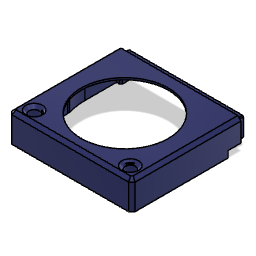
Custom_fan_TeslaK20xm_assembly (Autodesk Fusion 360 archive; units mm, degrees)
design "Case_top"
Autodesk Fusion 360 part; units mm, degrees
note: some values were not read from the file. Set by a fixed rule: which face or edge a step refers to.
sketch "Sketch1" plane through (0, 0, 0) normal (0, 1, 0) x (1, 0, 0)
  line L0 (48, -42.5) -> (-48, -42.5)
  line L1 (-48, -42.5) -> (-48, 42.5)
  line L2 (-48, 42.5) -> (48, 42.5)
  line L3 (48, 42.5) -> (48, -42.5)
  line L4 (48, -42.5) -> (-48, 42.5) construction
  line L5 (-48, -42.5) -> (48, 42.5) construction
  dimension "d1" = 96
  dimension "d2" = 85
  constraint horizontal L0
  constraint perpendicular L0 L1
  constraint parallel L0 L2
  constraint parallel L1 L3
  constraint coincident L4 origin
  constraint coincident L5 origin
  measures "d1" distance of L1.end L2.end
  measures "d2" distance of L0.end L1.end
extrude "Extrude1" add sketch "Sketch1" along normal blind 22.4
sketch "Sketch3" plane through (0, 22.4, 0) normal (0, 1, 0) x (-1, 0, 0)
  line L0 (-48, -42.5) -> (48, -42.5)
  line L1 (48, -42.5) -> (48, 42.5)
  line L2 (48, 42.5) -> (-48, 42.5)
  line L3 (-48, 42.5) -> (-48, -42.5)
  line L4 (48, -42.5) -> (-48, 42.5) construction
  line L5 (-48, -42.5) -> (48, 42.5) construction
  line L6 (0, 0) -> (48, 0) construction
  line L7 (0, 0) -> (0, -42.5) construction
  circle A0 centre (37.4349, 33.1455) radius 4
  circle A1 centre (37.4349, -33.1455) radius 4
  circle A2 centre (-37.4349, -33.1455) radius 4
  circle A3 centre (-37.4349, 33.1455) radius 4
  dimension "d7" = 8
  dimension "d17" = 50
  constraint coincident L0.end L1.start
  constraint coincident L2.end L3.start
  constraint coincident L0.start L3.end
  constraint coincident L1.end L2.start
  constraint coincident L6.start L7.start
  constraint midpoint L1 L6.end
  constraint midpoint L0 L7.end
  constraint coincident L5 A0.centre
  constraint symmetric L6 A0 A1
  constraint symmetric L7 A0 A3
  constraint symmetric L7 A1 A2
  measures "d7" diameter of A0
  measures "d17" distance of L6.start A0.centre
extrude "Extrude2" cut sketch "Sketch3" against normal up to surface (20.9 mm away) contours A0 | A3
chamfer "Chamfer2" distance 2.5 angle 45 2 edges at (-48, 11.2, 42.5) (48, 11.2, 42.5)
sketch "Sketch4" plane through (0, 22.4, 0) normal (0, 1, 0) x (-1, 0, 0)
  line L0 (-48, 40) -> (-48, -42.5)
  line L1 (-48, -42.5) -> (48, -42.5)
  line L2 (48, -42.5) -> (48, 40)
  line L3 (45.5, 42.5) -> (-45.5, 42.5)
  circle A0 centre (37.4349, 33.1455) radius 4
  circle A1 centre (-37.4349, 33.1455) radius 4
  circle A2 centre (0, 0) radius 34
  line L4 (-45.5, 42.5) -> (-48, 40)
  line L5 (48, 40) -> (45.5, 42.5)
  dimension "d11" = 68
  constraint coincident A2.centre origin
  measures "d11" diameter of A2
chamfer "Chamfer1" distance 2.5 angle 45 7 edges at (-48, 22.4, -1.25) (-46.75, 22.4, 41.25) (0, 22.4, 42.5) (46.75, 22.4, 41.25) (48, 22.4, -1.25) (-33.7056, 22.4, 34.592) (41.1642, 22.4, 34.592)
shell "Shell1" thickness 1.5 removed faces 2 at (-15.1667, 0, -14.1667) at (-15.1667, 7.4667, -42.5)
extrude "Extrude3" cut sketch "Sketch4" against normal through all contours A2
sketch "Sketch5" plane through (0, 0, 0) normal (0, -1, 0) x (1, 0, 0)
  circle A0 centre (-37.4349, 33.1455) radius 2.25
  line L0 (0, 0) -> (9, 0) construction
  line L1 (0, 0) -> (0, 1) construction
  line L2 (0, 1) -> (0, 8) construction
  circle A1 centre (37.4349, 33.1455) radius 2.25
  circle A2 centre (37.4349, 33.1455) radius 5.5
  line L3 (46.5, 39.3787) -> (46.5, -42.5)
  line L4 (46.5, -42.5) -> (48, -42.5)
  line L5 (48, -42.5) -> (48, 40)
  line L6 (48, 40) -> (45.5, 42.5)
  line L7 (45.5, 42.5) -> (-45.5, 42.5)
  line L8 (-45.5, 42.5) -> (-48, 40)
  line L9 (-48, 40) -> (-48, -42.5)
  line L10 (-48, -42.5) -> (-46.5, -42.5)
  line L11 (-46.5, -42.5) -> (-46.5, 39.3787)
  line L12 (-46.5, 39.3787) -> (-44.8787, 41)
  line L13 (-44.8787, 41) -> (44.8787, 41)
  line L14 (44.8787, 41) -> (46.5, 39.3787)
  circle A3 centre (-37.4349, 33.1455) radius 5.5
  dimension "d13" = 4.5
  constraint coincident L0.start L1.start
  constraint horizontal L0
  constraint perpendicular L0 L1
  constraint perpendicular L0 L2
  constraint symmetric A0 L2 A1
  measures "d13" diameter of A0
extrude "Extrude4" cut sketch "Sketch5" against normal through all contours A0 | A1
sketch "Sketch6" plane through (0, 0, 0) normal (0, -1, 0) x (1, 0, 0)
  line L0 (46.5, 39.3787) -> (46.5, -42.5)
  line L1 (46.5, -42.5) -> (48, -42.5)
  line L2 (48, -42.5) -> (48, 40)
  line L3 (48, 40) -> (45.5, 42.5)
  line L4 (45.5, 42.5) -> (-45.5, 42.5)
  line L5 (-45.5, 42.5) -> (-48, 40)
  line L6 (-48, 40) -> (-48, -42.5)
  line L7 (-48, -42.5) -> (-46.5, -42.5)
  line L8 (-46.5, -42.5) -> (-46.5, 39.3787)
  line L9 (-46.5, 39.3787) -> (-44.8787, 41)
  line L10 (-44.8787, 41) -> (44.8787, 41)
  line L11 (44.8787, 41) -> (46.5, 39.3787)
  line L12 (48, -42.5) -> (12, -42.5)
  line L13 (12, -42.5) -> (12, -41.1913)
  spline S0 degree 5 poles (14.495, -37.8387) (15.594, -37.5093) (17.7608, -36.7724) (20.9168, -35.4332) (24.9264, -33.1775) (29.5475, -29.5535) (33.7057, -25.1004) (37.3381, -19.8036) (40.4311, -13.6982) (43.0138, -6.8584) (45.1276, 0.6384) (46.4759, 7.1092) (47.3069, 12.2099) (47.7821, 15.7186) (48, 17.5) knots 0 0 0 0 0 0 0.1 0.2 0.3 0.4 0.5 0.6 0.7 0.8 0.9 1 1 1 1 1 1
  line L14 (48, 17.5) -> (48, -42.5)
  arc A0 (14.495, -37.8387) -> (12, -41.1913) centre (15.5, -41.1913) ccw
  line L15 (46.5, -41) -> (13.5092, -41)
  arc A1 (14.9257, -39.2756) -> (13.5092, -41) centre (15.5, -41.1913) ccw
  spline S1 degree 3 poles (14.9257, -39.2756) (22.097, -37.1258) (28.5847, -33.0615) (33.8097, -26.9591) (38.0341, -22.0255) (41.3619, -15.7498) (43.8832, -8.4629) (44.8686, -5.6148) (45.7368, -2.6127) (46.5, 0.5227) knots 0 0 0 0 0.377112 0.377112 0.377112 0.682001 0.682001 0.682001 0.801168 0.801168 0.801168 0.801168
  line L16 (46.5, 0.5227) -> (46.5, -41)
  circle A2 centre (0, 0) radius 44.4282 construction
  arc A3 (44.3977, -1.6437) -> (17.1132, 41) centre (0, 0) ccw
  arc A4 (45.8967, -1.6992) -> (17.691, 42.3843) centre (0, 0) ccw
  arc A5 (-17.1132, 41) -> (-44.4282, 0.0027) centre (0, 0) ccw
  line L17 (-44.8787, 38.7071) -> (-44.8787, -42.5)
  arc A6 (-17.691, 42.3843) -> (-45.9282, 0.0027) centre (0, 0) ccw
  line L18 (-44.4281, 0.0027) -> (-46.5, 0.0027)
  line L19 (-44.4281, 0.0027) -> (-44.4282, -1.4973)
  line L20 (-44.4282, -1.4973) -> (-46.5, -1.4973)
  point P0 (12, -38.5)
  point P1 (35, -23)
  dimension "d21" = 4
  dimension "d22" = 60
  dimension "d23" = 3.5
  dimension "d24" = 1.5
  dimension "d28" = 1.5
  dimension "d29" = 1.5
  dimension "d32" = 1.5
  constraint coincident L1.end L2.start
  constraint perpendicular L2 L12
  constraint perpendicular L12 L13
  constraint coincident L2 S0.end
  constraint perpendicular L1 L14
  constraint coincident P0 L13
  constraint tangent L13 A0
  constraint tangent S0 A0
  constraint coincident A2.centre A3.centre
  constraint coincident A2 A3.end
  constraint coincident S0 A3.start
  constraint coincident A2 A3.start
  constraint coincident L10 A3.end
  constraint coincident A2 L18.start
  constraint coincident A2 A5.start
  constraint coincident L10 A5.start
  constraint horizontal L18
  constraint tangent A2 L19
  constraint coincident L8 L20.end
  constraint perpendicular L8 L20
  measures "d21" distance of L12.end P0
  measures "d22" distance of L1.end S0.end
  measures "d23" radius of A0
  measures "d32" vertical distance of L18.start L19.end
extrude "Extrude6" add sketch "Sketch6" against normal up to surface (20.9 mm away) contours L10 S0 A3 A4 | L10 A5 L17 A6 L18
extrude "Extrude5" add sketch "Sketch6" against normal up to surface (20.9 mm away) contours L0 L12 L13 S0 A0 L15 A1 S1 | L17 L18 L19 L20 | L8 L17 L18 L20
fillet "Fillet3" radius 48 1 edges at (-46.5, 9.6393, -1.4973)
fillet "Fillet4" radius 20 3 edges at (-17.1132, 9.6393, 41) (17.1132, 9.6393, 41) (44.3977, 10.45, -1.6437)
sketch "Sketch7" plane through (48, 0, 0) normal (1, 0, 0) x (0, 0, -1)
  line L0 (42.5, 19.9) -> (-40, 19.9)
  line L1 (-40, 19.9) -> (-40, 0)
  line L2 (-40, 0) -> (42.5, 0)
  line L3 (42.5, 0) -> (42.5, 19.9)
  line L4 (42.5, 0) -> (32.5, 0)
  line L5 (32.5, 0) -> (32.5, 5)
  line L6 (32.5, 5) -> (42.5, 5)
  line L7 (42.5, 5) -> (42.5, 0)
  dimension "d37" = 10
  dimension "d38" = 5
  constraint horizontal L4
  constraint vertical L5
  constraint horizontal L6
  constraint vertical L7
  constraint coincident L2.end L3.start
  measures "d37" distance of L2.end L4.end
  measures "d38" distance of L2.end L6.end
extrude "Extrude7" cut sketch "Sketch7" against normal up to surface (36 mm away) contours L2 L3 L4 L5 L6 L7
sketch "Sketch8" plane through (0, 0, -42.5) normal (0, 0, -1) x (-1, 0, 0)
  line L0 (-48, 5) -> (-12, 5)
  line L1 (-12, 5) -> (-12, 20.9)
  line L2 (-12, 20.9) -> (44.8787, 20.9)
  line L3 (44.8787, 20.9) -> (46.5, 19.2787)
  line L4 (46.5, 19.2787) -> (46.5, 0)
  line L5 (46.5, 0) -> (48, 0)
  line L6 (48, 0) -> (48, 19.9)
  line L7 (48, 19.9) -> (45.5, 22.4)
  line L8 (45.5, 22.4) -> (-45.5, 22.4)
  line L9 (-45.5, 22.4) -> (-48, 19.9)
  line L10 (-48, 19.9) -> (-48, 5)
  line L11 (-45, 5) -> (-45, 18.6574)
  line L12 (-45, 18.6574) -> (-44.2574, 19.4)
  line L13 (-44.2574, 19.4) -> (44.2574, 19.4)
  line L14 (44.2574, 19.4) -> (45, 18.6574)
  line L15 (45, 18.6574) -> (45, 0)
  line L16 (43, 0) -> (45, 0)
  line L17 (45, 0) -> (46.5, 0)
  line L18 (-12, 19.4) -> (-12, 20.9)
  line L19 (44.8787, 20.9) -> (46.5, 19.2787)
  line L20 (46.5, 0) -> (46.5, 19.2787)
  line L21 (44.8787, 20.9) -> (-12, 20.9)
  line L22 (-43, 5) -> (-43, 17.4)
  line L23 (-43, 17.4) -> (43, 17.4)
  line L24 (43, 17.4) -> (43, 0)
  dimension "d41" = 3
  dimension "d42" = 3
  dimension "d43" = 3
  dimension "d45" = 3
  dimension "d46" = 3
  dimension "d47" = 2
  constraint coincident L0 L11.start
  constraint perpendicular L0 L11
  constraint parallel L2 L13
  constraint perpendicular L13 L15
  constraint parallel L9 L12
  constraint perpendicular L15 L16
  constraint coincident L4.end L5.start
  constraint perpendicular L4 L17
  constraint coincident L13 L18.start
  constraint coincident L1 L18.start
  constraint coincident L1.end L2.start
  constraint coincident L2.end L3.start
  constraint coincident L3.end L4.start
  measures "d41" distance of L6 L15
  measures "d42" distance of L7 L14
  measures "d43" distance of L8 L13
  measures "d45" distance of L9 L12
  measures "d46" distance of L10 L11
extrude "Extrude8" add sketch "Sketch8" along normal blind 5 contours L0 L1 L11 L12 L13 L22 L23 | L1 L13 L14 L15 L16 L23 L24
extrude "Extrude9" add sketch "Sketch8" against normal blind 2.5 contours L1 L13 L14 L15 L16 L23 L24 | L1 L2 L3 L4 L13 L14 L15 L17 L18 L19 L20 L21
chamfer "Chamfer3" distance 1.1 angle 45 2 edges at (-15.5, 17.4, -40) (-43, 8.7, -40)

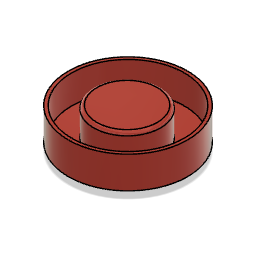
design "Fan_AVC_BASA0725R2U"
Autodesk Fusion 360 part; units mm, degrees
sketch "Sketch1" plane through (0, 0, 0) normal (0, 1, 0) x (1, 0, 0)
  circle A0 centre (0, 0) radius 21.362
  line L0 (0, 0) -> (21.362, 0)
  circle A1 centre (21.362, 0) radius 1.25
  circle A2 centre (-10.681, 18.5) radius 1.25
  circle A3 centre (-10.681, -18.5) radius 1.25
  line L1 (-10.681, 18.5) -> (21.362, 0) construction
  line L2 (-14.1333, 19.2835) -> (-14.1333, -19.2835)
  line L3 (-9.6333, -21.8816) -> (23.7667, -2.5981)
  line L4 (23.7667, 2.5981) -> (-9.6333, 21.8816)
  line L5 (-14.1333, 24.4797) -> (7.0667, -12.2398) construction
  line L6 (28.2667, 0) -> (-14.1333, 0) construction
  line L7 (-14.1333, -24.4797) -> (7.0667, 12.2398) construction
  arc A4 (-9.6333, 21.8816) -> (-14.1333, 19.2835) centre (-11.1333, 19.2835) ccw
  arc A5 (23.7667, -2.5981) -> (23.7667, 2.5981) centre (22.2667, 0) ccw
  arc A6 (-14.1333, -19.2835) -> (-9.6333, -21.8816) centre (-11.1333, -19.2835) ccw
  line L8 (25.2667, 13) -> (25.2667, -18) construction
  line L9 (-14.1333, -5) -> (-24.1333, -5)
  line L10 (-24.1333, -5) -> (-24.1333, 5)
  line L11 (-24.1333, 5) -> (-14.1333, 5)
  line L12 (-14.1333, 5) -> (-14.1333, -5)
  line L13 (-14.1333, -5) -> (-24.1333, 5) construction
  line L14 (-24.1333, -5) -> (-14.1333, 5) construction
  point P0 (-19.1333, 0)
  dimension "d1" = 2.5
  dimension "d3" = 360
  dimension "d4" = 37
  dimension "d6" = 60
  dimension "d7" = 60
  dimension "d8" = 3
  dimension "d9" = 39.4
  dimension "d12" = 10
  dimension "d13" = 10
  constraint coincident A0.centre L0.start
  constraint coincident A0 L0.end
  constraint horizontal L0
  constraint coincident L0.end A1.centre
  constraint coincident A2.centre L1.start
  constraint vertical L2
  constraint coincident L3 L5.end
  constraint perpendicular L3 L5
  constraint coincident L2 L6.end
  constraint perpendicular L2 L6
  constraint coincident L4 L7.end
  constraint perpendicular L4 L7
  constraint coincident L7 A0.centre
  constraint coincident L5 A0.centre
  constraint coincident L2 L5.start
  constraint coincident L5.start L4
  constraint tangent L2 A4
  constraint tangent L4 A4
  constraint coincident L6.start L4
  constraint coincident L6.start L3
  constraint tangent L4 A5
  constraint tangent L3 A5
  constraint equal A4 A5
  constraint coincident L7.start L3
  constraint coincident L7.start L2
  constraint tangent L3 A6
  constraint tangent L2 A6
  constraint equal A4 A6
  constraint vertical L8
  constraint tangent A5 L8
  constraint horizontal L9
  constraint perpendicular L9 L10
  constraint parallel L9 L11
  constraint parallel L10 L12
  constraint coincident L2 L9.start
  constraint coincident L13 P0
  constraint coincident L14 P0
  measures "d1" diameter of A1
  measures "d4" distance of A2.centre L0.end
  measures "d6" angle of L2 L3
  measures "d7" angle of L2 L4
  measures "d8" radius of A4
  measures "d9" distance of L2 L8
  measures "d12" distance of L9.start L9.end
  measures "d13" distance of L9.end L10.end
extrude "Extrude1" add sketch "Sketch1" along normal blind 1.2 contours A0 A1 A2 A3 L2 L3 L4 L12 | A0 A1 L3 L4 A5 | A0 A2 L2 L4 A4 | A0 A3 L2 L3 A6 | A0 L2 L9 L11 L12 | A0 L9 L10 L11 makes body 1
ref_plane "WorkPlane1" through (0.5667, 4.5, 0) normal (0, 1, 0) x (1, 0, 0)
sketch "Sketch2" plane through (0.5667, 4.5, 0) normal (0, 1, 0) x (1, 0, 0)
  circle A0 centre (0, 0) radius 37.5
  dimension "d15" = 75
  constraint coincident A0.centre origin
  measures "d15" diameter of A0
extrude "Extrude2" add sketch "Sketch2" along normal blind 20 separate body makes body 2
shell "Shell1" thickness 2 removed faces 1 at (5.273, 24.5, -13.499) on bodies 2
sketch "Sketch3" plane through (0, 6.5, 0) normal (0, 1, 0) x (-1, 0, 0)
  circle A0 centre (-0.5667, 0) radius 35.5
  circle A1 centre (0, 0) radius 21
  dimension "d19" = 42
  constraint coincident A1.centre origin
  measures "d19" diameter of A1
extrude "Extrude3" add sketch "Sketch3" along normal up to surface (18 mm away) contours A1 bodies 2
fillet "Fillet1" radius 2 1 edges at (19.5789, 24.5, 7.5939) on bodies 2

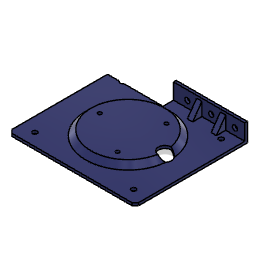
design "Case_bottom"
Autodesk Fusion 360 part; units mm, degrees
sketch "Sketch1" plane through (0, 0, 0) normal (0, 0, 1) x (1, 0, 0)
  line L0 (0, 0) -> (54, 0)
  line L1 (54, 0) -> (54, 14)
  line L2 (54, 14) -> (0, 14)
  line L3 (0, 14) -> (0, 0)
  line L4 (0, 7) -> (54, 7) construction
  circle A0 centre (46.5, 7) radius 1.9
  circle A1 centre (28.5, 7) radius 1.9
  circle A2 centre (10.5, 7) radius 1.9
  dimension "d1" = 54
  dimension "d2" = 14
  dimension "d3" = 3.8
  dimension "d4" = 3.8
  dimension "d5" = 3.8
  dimension "d6" = 7.5
  dimension "d7" = 18
  dimension "d8" = 18
  constraint horizontal L0
  constraint vertical L1
  constraint horizontal L2
  constraint vertical L3
  constraint coincident L0.start L3.end
  constraint midpoint L3 L4.start
  constraint midpoint L1 L4.end
  constraint coincident L4 A0.centre
  constraint coincident L4 A1.centre
  constraint coincident L4 A2.centre
  measures "d1" distance of L0.start L0.end
  measures "d2" distance of L0.start L2.end
  measures "d3" diameter of A0
  measures "d4" diameter of A1
  measures "d5" diameter of A2
  measures "d6" distance of L1 A0.centre
  measures "d7" distance of A0.centre A1.centre
  measures "d8" distance of A1.centre A2.centre
extrude "Extrude1" add sketch "Sketch1" along normal blind 2
sketch "Sketch2" plane through (0, 0, 0) normal (0, -1, 0) x (1, 0, 0)
  line L0 (0, 0) -> (54, 0)
  line L1 (54, 0) -> (54, 2)
  line L2 (54, 2) -> (0, 2)
  line L3 (0, 2) -> (0, 0)
  line L4 (54, 0) -> (-42, 0)
  line L5 (-42, 0) -> (-42, 85)
  line L6 (-42, 85) -> (54, 85)
  line L7 (54, 85) -> (54, 0)
  dimension "d11" = 96
  dimension "d14" = 85
  constraint horizontal L4
  constraint vertical L5
  constraint horizontal L6
  constraint vertical L7
  constraint coincident L0.end L1.start
  measures "d11" distance of L5.end L6.end
  measures "d14" distance of L4.end L5.end
extrude "Extrude2" add sketch "Sketch2" against normal blind 2
sketch "Sketch3" plane through (0, 2, 0) normal (0, 1, 0) x (-1, 0, 0)
  line L0 (-54, 2) -> (0, 2)
  line L1 (0, 2) -> (0, 0)
  line L2 (0, 0) -> (42, 0)
  line L3 (42, 0) -> (42, 85)
  line L4 (42, 85) -> (-54, 85)
  line L5 (-54, 85) -> (-54, 2)
  line L6 (-54, 85) -> (42, 0) construction
  line L7 (42, 85) -> (-54, 0) construction
  circle A0 centre (-6, 42.5) radius 21.362 construction
  circle A1 centre (-16.681, 24) radius 1.35
  circle A2 centre (-16.681, 61) radius 1.35
  circle A3 centre (15.362, 42.5) radius 1.35
  line L8 (-16.681, 24) -> (-16.681, 61) construction
  line L9 (15.362, 42.5) -> (-6, 42.5) construction
  line L10 (15.362, 42.5) -> (-16.681, 24) construction
  circle A4 centre (-34, 42.5) radius 5
  circle A5 centre (31.4349, 75.6455) radius 1.75
  line L11 (-6, 42.5) -> (-6, 21.138) construction
  circle A6 centre (31.4349, 9.3545) radius 1.75
  circle A7 centre (-43.4349, 9.3545) radius 1.75
  circle A8 centre (-43.4349, 75.6455) radius 1.75
  line L12 (-6, 42.5) -> (-34, 42.5) construction
  circle A9 centre (-6, 42.5) radius 28
  point P0 (-54, 0)
  point P1 (-6, 42.5)
  dimension "d15" = 2.7
  dimension "d16" = 2.7
  dimension "d17" = 2.7
  dimension "d18" = 37
  dimension "d20" = 37
  dimension "d22" = 28
  dimension "d23" = 10
  dimension "d26" = 3.5
  dimension "d27" = 50
  constraint coincident L4.end L5.start
  constraint coincident L2.end L3.start
  constraint coincident L3.end L4.start
  constraint coincident P0 L7.end
  constraint midpoint L6 P1
  constraint coincident P1 A0.centre
  constraint coincident A0 A1.centre
  constraint coincident A0 A2.centre
  constraint coincident A0 A3.centre
  constraint coincident A1.centre L8.start
  constraint coincident A2.centre L8.end
  constraint vertical L8
  constraint coincident A3.centre L9.start
  constraint horizontal L9
  constraint coincident L7 A5.centre
  constraint coincident A0 L11.end
  constraint perpendicular L9 L11
  constraint symmetric L9 A5 A6
  constraint symmetric A5 L11 A8
  constraint symmetric L11 A6 A7
  constraint coincident A4.centre L12.end
  constraint horizontal L12
  constraint coincident A4.centre A9
  measures "d15" diameter of A1
  measures "d16" diameter of A2
  measures "d17" diameter of A3
  measures "d18" distance of A1.centre A2.centre
  measures "d20" distance of A3.centre A1.centre
  measures "d22" distance of P1 A4.centre
  measures "d23" diameter of A4
  measures "d26" diameter of A5
  measures "d27" distance of P1 A5.centre
extrude "Extrude4" add sketch "Sketch3" along normal blind 4 contours A4 A9 picked at (-6, 42.5)
extrude "Extrude3" cut sketch "Sketch3" against normal through all contours A1 | A2 | A3 | A4 A9 | A4 A9 | A5 | A6 | A7 | A8 picked at (-32.3002, 42.5) picked at (-35.6292, 42.3798)
chamfer "Chamfer3" distance 2.5 angle 45 2 edges at (-42, 1, 85) (54, 1, 85)
chamfer "Chamfer1" distance 4 angle 45 1 edges at (-22, 2, 42.5)
sketch "Sketch4" plane through (0, 0, 0) normal (0, -1, 0) x (1, 0, 0)
  line L0 (51.5, 85) -> (-39.5, 85)
  line L1 (-42, 82.5) -> (-42, 0)
  line L2 (-42, 0) -> (54, 0)
  line L3 (54, 0) -> (54, 82.5)
  circle A0 centre (-31.4349, 9.3545) radius 1.75
  circle A1 centre (16.681, 61) radius 1.35
  circle A2 centre (-15.362, 42.5) radius 1.35
  circle A3 centre (43.4349, 9.3545) radius 1.75
  circle A4 centre (-31.4349, 75.6455) radius 1.75
  circle A5 centre (34, 42.5) radius 5
  circle A6 centre (16.681, 24) radius 1.35
  circle A7 centre (43.4349, 75.6455) radius 1.75
  line L4 (6, 0) -> (6, 85) construction
  line L5 (6, 42.5) -> (54, 42.5) construction
  circle A8 centre (6, 42.5) radius 28
  line L6 (54, 82.5) -> (51.5, 85)
  line L7 (-39.5, 85) -> (-42, 82.5)
  dimension "d31" = 56
  constraint midpoint L2 L4.start
  constraint midpoint L0 L4.end
  constraint midpoint L4 L5.start
  constraint coincident L3 L5.end
  constraint perpendicular L3 L5
  constraint coincident L5.start A8.centre
  measures "d31" diameter of A8
extrude "Extrude5" cut sketch "Sketch4" against normal blind 4 contours A5 A8 picked at (6, 42.5)
chamfer "Chamfer2" distance 4 angle 45 1 edges at (-22, 0, 42.5)
sketch "Sketch5" plane through (0, 0, 2) normal (0, 0, 1) x (1, 0, 0)
  line L0 (0, 2) -> (54, 2)
  line L1 (54, 2) -> (54, 14)
  line L2 (54, 14) -> (0, 14)
  line L3 (0, 14) -> (0, 2)
  circle A0 centre (46.5, 7) radius 1.9
  circle A1 centre (28.5, 7) radius 1.9
  circle A2 centre (10.5, 7) radius 1.9
  line L4 (10.5, 7) -> (28.5, 7) construction
  line L5 (28.5, 7) -> (46.5, 7) construction
  line L6 (21.5, 2) -> (17.5, 2)
  line L7 (17.5, 2) -> (17.5, 12)
  line L8 (17.5, 12) -> (21.5, 12)
  line L9 (21.5, 12) -> (21.5, 2)
  line L10 (21.5, 2) -> (17.5, 12) construction
  line L11 (17.5, 2) -> (21.5, 12) construction
  line L12 (39.5, 2) -> (35.5, 2)
  line L13 (35.5, 2) -> (35.5, 12)
  line L14 (35.5, 12) -> (39.5, 12)
  line L15 (39.5, 12) -> (39.5, 2)
  line L16 (39.5, 2) -> (35.5, 12) construction
  line L17 (35.5, 2) -> (39.5, 12) construction
  point P0 (19.5, 7)
  point P1 (37.5, 7)
  dimension "d36" = 4
  dimension "d37" = 4
  constraint coincident A2.centre L4.start
  constraint coincident A1.centre L4.end
  constraint coincident A0.centre L5.end
  constraint horizontal L6
  constraint perpendicular L6 L7
  constraint parallel L6 L8
  constraint parallel L7 L9
  constraint coincident L10 P0
  constraint coincident L11 P0
  constraint midpoint L4 P0
  constraint horizontal L12
  constraint perpendicular L12 L13
  constraint parallel L12 L14
  constraint parallel L13 L15
  constraint coincident L0 L12.start
  constraint coincident L16 P1
  constraint coincident L17 P1
  constraint midpoint L5 P1
  constraint collinear L6 L12
  measures "d36" distance of L7.end L8.end
  measures "d37" distance of L13.end L14.end
extrude "Extrude6" add sketch "Sketch5" along normal blind 7 contours L0 L6 L7 L8 L9 | L0 L12 L13 L14 L15
chamfer "Chamfer4" distance 10 distance2 7 2 edges at (19.5, 12, 9) (37.5, 12, 9) measured on face at (20.1667, 5.3333, 9) measured on face at (36.8333, 5.3333, 9)
sketch "Sketch7" plane through (0, 2, 0) normal (0, 1, 0) x (-1, 0, 0)
  line L0 (-35.5, 9) -> (-35.5, 2)
  line L1 (-35.5, 2) -> (-21.5, 2)
  line L2 (0, 2) -> (0, 0)
  line L3 (0, 0) -> (42, 0)
  line L4 (42, 0) -> (42, 82.5)
  line L5 (42, 82.5) -> (39.5, 85)
  line L6 (39.5, 85) -> (-51.5, 85)
  line L7 (-51.5, 85) -> (-54, 82.5)
  line L8 (-54, 82.5) -> (-54, 2)
  line L9 (-54, 2) -> (-39.5, 2)
  line L10 (-39.5, 2) -> (-39.5, 9)
  arc A0 (-37.8393, 39.2969) -> (-37.8393, 45.7031) centre (-6, 42.5) ccw
  arc A1 (-37.8393, 45.7031) -> (-37.8393, 39.2969) centre (-34, 42.5) ccw
  circle A2 centre (-43.4349, 75.6455) radius 1.75
  circle A3 centre (31.4349, 75.6455) radius 1.75
  circle A4 centre (-43.4349, 9.3545) radius 1.75
  circle A5 centre (31.4349, 9.3545) radius 1.75
  line L11 (42, 0) -> (0, 0)
  line L12 (0, 0) -> (0, 10)
  line L13 (0, 10) -> (42, 10)
  line L14 (42, 10) -> (42, 0)
  line L15 (-21.5, 2) -> (-21.5, 9)
  line L16 (-17.5, 9) -> (-17.5, 2)
  line L17 (-21.5, 9) -> (-17.5, 9)
  line L18 (-17.5, 2) -> (0, 2)
  line L19 (-39.5, 9) -> (-35.5, 9)
  dimension "d49" = 10
  constraint horizontal L11
  constraint vertical L12
  constraint horizontal L13
  constraint vertical L14
  constraint coincident L3.end L4.start
  constraint collinear L2 L12
  measures "d49" distance of L3.end L13.end
extrude "Extrude7" cut sketch "Sketch7" against normal through all contours L2 L3 L4 A5 L11 L12 L13 L14
